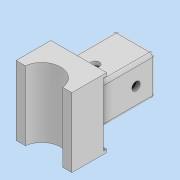
# Autodesk Inventor part: 5_Connettore_sup_inf
Saved by Autodesk Inventor 2020 (Build 240168000, 168)
## iProperties
Created: 2019-10-13
Part Number: 5_Connettore_sup_inf
Material: Generico
Document SubType Name: Modeling
Designer: socci
Density: 1 g/cm^3
Appearance: Default
Author: socci
Autodesk Inventor part; units mm, degrees
ref_plane "YZ Plane" through (0, 0, 0) normal (1, 0, 0) x (0, 1, 0)
ref_plane "XZ Plane" through (0, 0, 0) normal (0, 1, 0) x (-1, 0, 0)
ref_plane "XY Plane" through (0, 0, 0) normal (0, 0, 1) x (1, 0, 0)
sketch "Schizzo1" plane through (0, 0, 0) normal (0, 0, 1) x (1, 0, 0)
  line L0 (9, 6) -> (9, -6)
  line L1 (6, -9) -> (-6, -9)
  line L2 (-9, -6) -> (-9, 6)
  line L3 (-6, 9) -> (6, 9)
  arc A0 (-6, 9) -> (-9, 6) centre (-6, 6) ccw
  arc A1 (-9, -6) -> (-6, -9) centre (-6, -6) ccw
  arc A2 (6, -9) -> (9, -6) centre (6, -6) ccw
  arc A3 (9, 6) -> (6, 9) centre (6, 6) ccw
  point P0 (0, 0)
  point P1 (0, 0)
  point P2 (9, 9)
  point P3 (9, -9)
  point P4 (-9, -9)
  point P5 (-9, 9)
  dimension "d0" = 18
  dimension "d72" = 3
  constraints: 8 end point, 8 point on circle, 8 point on line, 8 tangent, 4 centre point, 3 equal radius, 1 coincident, 9 other
  measures "d0" distance of point (9, 9) point (9, -9)
  measures "d72" radius of A0
extrude "Estrusione1" add sketch "Schizzo1" against normal blind 40
sketch "Schizzo2" plane through (0, 0, 0) normal (0, 0, 1) x (1, 0, 0)
  line L0 (18.5, -23) -> (-18.5, -23)
  line L1 (-18.5, -23) -> (-18.5, 23)
  line L2 (-18.5, 23) -> (18.5, 23)
  line L3 (18.5, 23) -> (18.5, -23)
  line L4 (18.5, -23) -> (-18.5, 23) construction
  line L5 (-18.5, -23) -> (18.5, 23) construction
  point P0 (0, 0)
  dimension "d3" = 46
  dimension "d4" = 37
  constraints: 12 end point, 3 midpoint, 2 parallel, 1 horizontal, 1 perpendicular
  measures "d3" distance of L0.end L1.end
  measures "d4" distance of L1.end L2.end
extrude "Estrusione2" add sketch "Schizzo2" along normal blind 21
sketch "Schizzo3" plane through (-18.5, 23, 0) normal (0, 1, 0) x (1, 0, 0)
  line L0 (18.5, 0) -> (18.5, -22.5)
  line L1 (18.5, 0) -> (41, 0) construction
  circle A0 centre (18.5, -22.5) radius 12.5
  dimension "d7" = 22.5
  dimension "d8" = 90
  dimension "d9" = 25
  constraints: 4 end point, 1 centre point, 1 coincident, 1 horizontal, 1 perpendicular, 1 vertical
  measures "d7" distance of L0.start L0.end
  measures "d8" angle of L0 L1
  measures "d9" diameter of A0
extrude "Estrusione3" cut sketch "Schizzo3" against normal blind 46
sketch "Schizzo7" plane through (-18.5, 23, 0) normal (0, 1, 0) x (1, 0, 0)
  arc A0 (30.9097, -21) -> (6.0903, -21) centre (18.5, -22.5) ccw projected
  line L0 (0, 0) -> (0, -22.5)
  circle A1 centre (18.5, -22.5) radius 18.5
  line L1 (18.5, 0) -> (4.5, 0)
  line L2 (37, 0) -> (0, 0) projected
  line L3 (18.5, 0) -> (32.5, 0) construction
  line L4 (4.5, 0) -> (4.5, -10.4066)
  point P0 (16.5, -34.839)
  point P1 (20.5, -34.839)
  dimension "d73" = 37
  dimension "d74" = 14
  dimension "d75" = 180
  dimension "d76" = 90
  constraints: 8 end point, 2 collinear, 1 coincident, 1 horizontal, 3 other
  measures "d74" distance of L1.start L1.end
  measures "d75" angle of L1 L3
  measures "d76" angle of L4 L1
extrude "Estrusione7" [suppressed]
sketch "Schizzo8" plane through (0, 23, 22.5) normal (0, 1, 0) x (1, 0, 0)
  line L0 (-6, 22.5) -> (6, 22.5) projected
  arc A0 (12.4097, 1.5) -> (-12.4097, 1.5) centre (0, 0) ccw projected
  circle A1 centre (0, 0) radius 18.5
  line L1 (0, 22.5) -> (14, 22.5)
  line L2 (0, 22.5) -> (14, 22.5) construction
  line L3 (14, 22.5) -> (14, 12.0934)
  line L4 (-18.5, 22.5) -> (18.5, 22.5) projected
  line L5 (14, 22.5) -> (18.5, 22.5)
  line L6 (18.5, 22.5) -> (18.5, 0)
  point P0 (-9, 22.5)
  point P1 (9, 22.5)
  point P2 (2, -12.339)
  point P3 (-2, -12.339)
  point P4 (-14, 22.5)
  dimension "d35" = 37
  dimension "d36" = 14
  dimension "d38" = 90
  constraints: 10 end point, 2 collinear, 2 horizontal, 2 point on circle, 1 centre point, 1 coincident, 1 perpendicular
  measures "d35" diameter of A1
  measures "d36" distance of L1.start L1.end
  measures "d38" angle of L1 L3
extrude "Estrusione8" [suppressed]
sketch "Schizzo14" plane through (0, 0, 0) normal (0, 0, -1) x (-1, 0, 0)
  line L0 (-11, 13) -> (11, 13)
  line L1 (13, 11) -> (13, -11)
  line L2 (11, -13) -> (-11, -13)
  line L3 (-13, -11) -> (-13, 11)
  arc A0 (11, -13) -> (13, -11) centre (11, -11) ccw
  arc A1 (-13, -11) -> (-11, -13) centre (-11, -11) ccw
  arc A2 (13, 11) -> (11, 13) centre (11, 11) ccw
  arc A3 (-11, 13) -> (-13, 11) centre (-11, 11) ccw
  line L4 (-9.382, 10.5) -> (9.382, 10.5)
  line L5 (10.5, 9.382) -> (10.5, -9.382)
  line L6 (9.382, -10.5) -> (-9.382, -10.5)
  line L7 (-10.5, -9.382) -> (-10.5, 9.382)
  arc A4 (-10.1273, 10.8333) -> (-10.8333, 10.1273) centre (-10.5, 10.5) ccw
  arc A5 (-10.1273, 10.8333) -> (-9.382, 10.5) centre (-9.382, 11.5) ccw
  arc A6 (-10.5, 9.382) -> (-10.8333, 10.1273) centre (-11.5, 9.382) ccw
  arc A7 (10.8333, 10.1273) -> (10.1273, 10.8333) centre (10.5, 10.5) ccw
  arc A8 (9.382, 10.5) -> (10.1273, 10.8333) centre (9.382, 11.5) ccw
  arc A9 (10.8333, 10.1273) -> (10.5, 9.382) centre (11.5, 9.382) ccw
  arc A10 (10.1273, -10.8333) -> (10.8333, -10.1273) centre (10.5, -10.5) ccw
  arc A11 (10.1273, -10.8333) -> (9.382, -10.5) centre (9.382, -11.5) ccw
  arc A12 (10.5, -9.382) -> (10.8333, -10.1273) centre (11.5, -9.382) ccw
  arc A13 (-10.8333, -10.1273) -> (-10.1273, -10.8333) centre (-10.5, -10.5) ccw
  arc A14 (-9.382, -10.5) -> (-10.1273, -10.8333) centre (-9.382, -11.5) ccw
  arc A15 (-10.8333, -10.1273) -> (-10.5, -9.382) centre (-11.5, -9.382) ccw
  point P0 (0, 0)
  point P1 (0, 0)
  point P2 (-10.5, 10.5)
  point P3 (10.5, 10.5)
  point P4 (10.5, -10.5)
  point P5 (-10.5, -10.5)
  point P6 (0, 0)
  point P7 (-13, 13)
  point P8 (13, 13)
  point P9 (13, -13)
  point P10 (-13, -13)
  point P11 (0, 0)
  point P12 (-10, 10.5)
  point P13 (-10.5, 10)
  point P14 (10.5, 10)
  point P15 (10, 10.5)
  point P16 (10, -10.5)
  point P17 (10.5, -10)
  point P18 (-10.5, -10)
  point P19 (-10, -10.5)
  dimension "d77" = 21
  dimension "d78" = 26
  dimension "d102" = 2
  dimension "d110" = 1
  dimension "d112" = 1
  dimension "d114" = 1
  dimension "d116" = 1
  constraints: 40 point on circle, 24 tangent, 16 centre point, 16 end point, 16 point on line, 5 equal radius, 3 coincident, 19 other
  measures "d77" distance of point (-10.5, -10.5) point (-10.5, 10.5)
  measures "d78" distance of point (-13, -13) point (-13, 13)
  measures "d102" radius of A2
  measures "d110" radius of A5
  measures "d112" radius of A8
  measures "d114" radius of A11
  measures "d116" radius of A14
extrude "Estrusione10" add sketch "Schizzo14" along normal blind 40
sketch "Schizzo15" plane through (-13, 13, 0) normal (0, 1, 0) x (1, 0, 0)
  line L0 (13, 0) -> (13, 13)
  line L1 (13, 0) -> (26, 0) construction
  dimension "d82" = 13
  dimension "d83" = 90
  constraints: 4 end point, 1 horizontal, 1 perpendicular, 1 vertical
  measures "d82" distance of L0.start L0.end
  measures "d83" angle of L1 L0
hole "Foro4" at (0, 13, -13) direction (0, -1, 0) diameter 5.5 depth 26 tip angle 118 clearance for "Vite a testa esagonale" size "M5" standard "ANSI - Profilo M Metrico"
sketch "Schizzo16" plane through (13, -11, 0) normal (1, 0, 0) x (0, 0, -1)
  line L0 (0, 11) -> (27, 11)
  line L1 (0, 11) -> (27, 11) construction
  dimension "d91" = 27
  dimension "d92" = 0
  constraints: 4 end point, 2 horizontal, 1 collinear
  measures "d91" distance of L0.start L0.end
  measures "d92" distance between parallel lines of L0 L1
hole "Foro5" at (13, 0, -27) direction (-1, 0, 0) diameter 5.5 depth 26 tip angle 118 clearance for "Vite a testa esagonale" size "M5" standard "ANSI - Profilo M Metrico"
fillet "Raccordo1" radius 2 1 edges at (0, -13, -40)
fillet "Raccordo2" radius 2 1 edges at (-9, 0, -40)
fillet "Raccordo3" radius 3 1 edges at (-13, 0, 0)
sketch "Schizzo17" plane through (0, 0, 0) normal (0, 0, -1) x (-1, 0, 0)
  point P0 (0, 0)
sketch "Schizzo18" plane through (0, 0, 0) normal (0, 0, -1) x (-1, 0, 0)
  line L0 (18.5, -23) -> (12.4097, -23) projected
  line L1 (18.5, 23) -> (18.5, -23) projected
  line L2 (-18.5, -23) -> (-18.5, 23) projected
  line L3 (18.5, -23) -> (-18.5, -23)
  line L4 (-18.5, -23) -> (-18.5, -21)
  line L5 (-18.5, -21) -> (18.5, -21)
  line L6 (18.5, -21) -> (18.5, -23)
  line L7 (12.4097, -23) -> (-12.4097, -23) projected
  line L8 (12.4097, 23) -> (18.5, 23) projected
  line L9 (18.5, 23) -> (-18.5, 23)
  line L10 (-18.5, 23) -> (-18.5, 21)
  line L11 (-18.5, 21) -> (18.5, 21)
  line L12 (18.5, 21) -> (18.5, 23)
  point P0 (0, 0)
  dimension "d104" = 2
  dimension "d105" = 2
  constraints: 16 end point, 4 parallel, 2 collinear, 2 perpendicular
  measures "d104" distance of L2.start L4.end
  measures "d105" distance of L10.end L2.end
extrude "Estrusione11" add sketch "Schizzo18" along normal blind 2 contours L0 L3 L2 L5 L1 | L11 L2 L9 L8 L1
